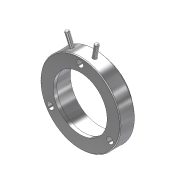
# Autodesk Inventor part: Part38
Saved by Autodesk Inventor 2011 (Build 150239000, 239)
## iProperties
Created: 2012-04-09
Part Number: Part38
Material: Steel
Document SubType Name: Modeling
Designer: jhanson2
Density: 7.85 g/cm^3
Author: jhanson2
Autodesk Inventor part; units mm, degrees
ref_plane "YZ Plane" through (0, 0, 0) normal (1, 0, 0) x (0, 1, 0)
sketch "Sketch1" plane through (0, 0, 0) normal (0, 0, 1) x (1, 0, 0)
  circle A0 centre (0, 0) radius 26.1938
  circle A1 centre (0, 0) radius 38.8938
  dimension "d0" = 77.7875
  dimension "d1" = 12.7
  constraints: 2 centre point, 2 coincident
  measures "d0" diameter of A1
  measures "d1" radial gap between concentric circles of A1 A0
extrude "Extrusion1" add sketch "Sketch1" along normal blind 14.5288
sketch "Sketch2" plane through (0, 0, 0) normal (0, 0, -1) x (-1, 0, 0)
  circle A0 centre (0, 0) radius 38.8938 projected
  circle A1 centre (0, 0) radius 28.575
  circle A2 centre (0, 0) radius 33.3375
  dimension "d5" = 4.7625
  dimension "d41" = 5.5563
  constraints: 2 centre point, 2 coincident
  measures "d5" radial gap between concentric circles of A1 A2
  measures "d41" radial gap between concentric circles of A2 A0
extrude "Extrusion2" add sketch "Sketch2" along normal blind 4.5212 contours A2
chamfer "Chamfer1" distance 0.7874 angle 45 1 edges at (33.3375, 0, -4.5212)
extrude "Extrusion3" cut sketch "Sketch2" against normal blind 11.1125 contours A1
sketch "Sketch3" plane through (0, 0, 14.5288) normal (0, 0, 1) x (1, 0, 0)
  circle A0 centre (0, 0) radius 38.8938 projected
  circle A1 centre (0, 33.3375) radius 3.175
  line L0 (0, 33.3375) -> (0, 0) construction
  dimension "d14" = 33.3375
  dimension "d15" = 6.35
  constraints: 2 end point, 1 centre point, 1 vertical
  measures "d14" distance of L0.start L0.end
  measures "d15" diameter of A1
extrude "Extrusion4" cut sketch "Sketch3" against normal blind 10.414 contours A1
pattern_circular "Circular Pattern1" count 3 over 360 about axis through (0, 0, 0) along (0, 0, 1) of "Extrusion4"
fillet "Fillet2" radius 0.7874 2 edges at (-38.8938, 0, 14.5288) (-38.8938, 0, 0)
sketch "Sketch4" plane through (0, 0, 14.5288) normal (0, 0, 1) x (1, 0, 0)
  circle A0 centre (0, 0) radius 26.1938 projected
  circle A1 centre (0, 33.3375) radius 3.175 projected
  circle A2 centre (-28.8711, -16.6687) radius 3.175 projected
  circle A3 centre (28.8711, -16.6688) radius 3.175 projected
  circle A4 centre (0, 0) radius 38.1064 projected
  line L0 (0, 0) -> (0, 33.3375) construction
  line L1 (8.1747, 37.2192) -> (10.5126, 50.4781) construction
  line L2 (0, 0) -> (8.9493, 50.7538) construction
  line L3 (5.048, 37.7705) -> (7.3859, 51.0295) construction
  line L4 (7.3859, 51.0295) -> (10.5126, 50.4781) construction
  line L5 (-13.4151, 35.6669) -> (-18.4691, 47.5734) construction
  line L6 (-16.3125, 34.3669) -> (-21.3917, 46.3328) construction
  line L7 (-21.3917, 46.3328) -> (-18.4691, 47.5734) construction
  line L8 (-19.9304, 46.9531) -> (0, 0) construction
  circle A5 centre (0, 46.0375) radius 6.35 projected
  dimension "d29" = 3.175
  dimension "d31" = 3.175
  dimension "d33" = 10
  dimension "d34" = 23
  constraints: 18 end point, 4 perpendicular, 3 point on circle, 2 midpoint, 2 parallel, 1 coincident
  measures "d29" distance between parallel lines of L1 L3
  measures "d31" distance between parallel lines of L5 L6
  measures "d33" angle of L2 L0
  measures "d34" angle of L0 L8
sketch "Sketch5" plane through (0, 0, 0) normal (0, 0, -1) x (-1, 0, 0)
  circle A0 centre (0, 0) radius 33.3375 projected
  circle A1 centre (0, 0) radius 38.1064 projected
  line L0 (19.9304, 46.9531) -> (0, 0) construction
  line L1 (0, 0) -> (-8.9493, 50.7538) construction
ref_plane "Work Plane1" through (0, 0, 14.5288) normal (-0.9848078, 0.1736482, 0) x (0.1736482, 0.9848078, 0)
ref_plane "Work Plane2" through (-19.9304, 46.9531, 0) normal (-0.9205049, -0.3907311, 0) x (0.3907311, -0.9205049, 0)
sketch "Sketch6" plane through (0, 0, 14.5288) normal (-0.9848078, 0.1736482, 0) x (0.1736482, 0.9848078, 0)
  line L0 (26.1938, 3.4163) -> (28.575, 3.4163) projected
  line L1 (26.1938, 0) -> (26.1938, 3.4163) projected
  line L2 (38.1064, 0) -> (26.1938, 0) projected
  arc A0 (38.1064, 0) -> (38.8938, 0.7874) centre (38.1064, 0.7874) ccw projected
  line L3 (38.8938, 13.7414) -> (38.8938, 0.7874) projected
  arc A1 (38.8938, 13.7414) -> (38.1064, 14.5288) centre (38.1064, 13.7414) ccw projected
  line L4 (33.3375, 14.5288) -> (38.1064, 14.5288) projected
  line L5 (33.3375, 18.2626) -> (33.3375, 14.5288) projected
  line L6 (32.5501, 19.05) -> (33.3375, 18.2626) projected
  line L7 (-33.3375, 18.2626) -> (-32.5501, 19.05) projected
  line L8 (-33.3375, 14.5288) -> (-33.3375, 18.2626) projected
  line L9 (-38.1064, 14.5288) -> (-33.3375, 14.5288) projected
  arc A2 (-38.1064, 14.5288) -> (-38.8938, 13.7414) centre (-38.1064, 13.7414) ccw projected
  line L10 (-38.8938, 0.7874) -> (-38.8938, 13.7414) projected
  arc A3 (-38.8938, 0.7874) -> (-38.1064, 0) centre (-38.1064, 0.7874) ccw projected
  line L11 (-26.1938, 0) -> (-38.1064, 0) projected
  line L12 (-26.1938, 3.4163) -> (-26.1938, 0) projected
  line L13 (-28.575, 3.4163) -> (-26.1938, 3.4163) projected
  line L14 (-38.8938, 5.28) -> (50.8, 5.28)
  line L15 (50.8, 5.28) -> (50.8, 7.2644)
  line L16 (-38.8938, 7.2644) -> (-38.8938, 5.28)
  arc A4 (50.8, 5.28) -> (52.7844, 7.2644) centre (50.8, 7.2644) ccw
  line L17 (50.8, 7.2644) -> (52.7844, 7.2644)
  line L18 (50.8, 7.2644) -> (-38.8938, 7.2644)
  line L19 (-38.8938, 7.2644) -> (35.5918, 7.2644)
  line L20 (35.5918, 7.2644) -> (35.5918, 5.28)
  line L21 (35.5918, 5.28) -> (-38.8938, 5.28)
  line L22 (-38.8938, 5.28) -> (-38.8938, 7.2644)
  line L23 (-26.1938, 1.7081) -> (26.1938, 1.7082) construction
  line L24 (0, 1.7081) -> (0, 14.5288) construction
  line L25 (28.575, 3.4163) -> (28.575, 19.05) projected
  line L26 (28.575, 19.05) -> (32.5501, 19.05) projected
  line L27 (-32.5501, 19.05) -> (-28.575, 19.05) projected
  line L28 (-28.575, 19.05) -> (-28.575, 3.4163) projected
  dimension "d35" = 3.9688
  dimension "d42" = 50.8
  constraints: 22 end point, 4 midpoint, 3 horizontal, 3 parallel, 3 perpendicular, 2 point on circle, 1 centre point, 1 collinear, 1 point on line, 1 tangent
  measures "d35" diameter of L14 L18
  measures "d42" distance from line of L24 L15.end
revolve "Revolution1" add sketch "Sketch6" angle 360 about axis through (8.8213, 50.0282, 7.2644) along (-0.1736482, -0.9848078, 0) contours L20 L18 L3 L14 | L3 L18 L15 L14 | L15 L17 A4
sketch "Sketch7" plane through (-19.9304, 46.9531, 0) normal (-0.9205049, -0.3907311, 0) x (0.3907311, -0.9205049, 0)
  line L0 (24.8142, 11.1125) -> (22.4329, 11.1125) projected
  line L1 (24.8142, 14.5288) -> (24.8142, 11.1125) projected
  line L2 (12.9016, 14.5288) -> (24.8142, 14.5288) projected
  arc A0 (12.9016, 14.5288) -> (12.1142, 13.7414) centre (12.9016, 13.7414) ccw projected
  line L3 (12.1142, 0.7874) -> (12.1142, 13.7414) projected
  arc A1 (12.1142, 0.7874) -> (12.9016, 0) centre (12.9016, 0.7874) ccw projected
  line L4 (17.6704, 0) -> (12.9016, 0) projected
  line L5 (17.6704, -3.7338) -> (17.6704, 0) projected
  line L6 (18.4578, -4.5212) -> (17.6704, -3.7338) projected
  line L7 (84.3454, -3.7338) -> (83.558, -4.5212) projected
  line L8 (84.3454, 0) -> (84.3454, -3.7338) projected
  line L9 (89.1143, 0) -> (84.3454, 0) projected
  arc A2 (89.1143, 0) -> (89.9017, 0.7874) centre (89.1143, 0.7874) ccw projected
  line L10 (89.9017, 13.7414) -> (89.9017, 0.7874) projected
  arc A3 (89.9017, 13.7414) -> (89.1143, 14.5288) centre (89.1143, 13.7414) ccw projected
  line L11 (77.2017, 14.5288) -> (89.1143, 14.5288) projected
  line L12 (77.2017, 11.1125) -> (77.2017, 14.5288) projected
  line L13 (79.5829, 11.1125) -> (77.2017, 11.1125) projected
  line L14 (89.9017, 7.2644) -> (0.2079, 7.2644)
  line L15 (0.2079, 7.2644) -> (0.2079, 9.2488)
  line L16 (0.2079, 9.2488) -> (89.9017, 9.2488)
  line L17 (89.9017, 9.2488) -> (89.9017, 7.2644)
  line L18 (89.9017, 7.2644) -> (14.9633, 7.2644)
  line L19 (14.9633, 7.2644) -> (14.9633, 9.2488)
  line L20 (14.9633, 9.2488) -> (89.9017, 9.2488)
  line L21 (89.9017, 9.2488) -> (89.9017, 7.2644)
  line L22 (0.2079, 7.2644) -> (-1.7764, 7.2644)
  arc A4 (0.2079, 9.2488) -> (-1.7764, 7.2644) centre (0.2079, 7.2644) ccw
  line L23 (51.0079, 0) -> (51.0079, 17.9555) construction
  line L24 (22.4329, 11.1125) -> (22.4329, -4.5212) projected
  line L25 (22.4329, -4.5212) -> (18.4578, -4.5212) projected
  line L26 (83.558, -4.5212) -> (79.5829, -4.5212) projected
  line L27 (79.5829, -4.5212) -> (79.5829, 11.1125) projected
  dimension "d39" = 3.9688
  dimension "d43" = 50.8
  constraints: 20 end point, 4 parallel, 4 perpendicular, 2 horizontal, 2 point on circle, 1 centre point, 1 collinear, 1 midpoint, 1 point on line, 1 tangent
  measures "d39" diameter of L16 L14
  measures "d43" distance from line of L23 L14.end
revolve "Revolution2" add sketch "Sketch7" angle 360 about axis through (15.197, -35.8019, 7.2644) along (-0.3907311, 0.9205049, 0) contours L19 L14 L3 L16 | L3 L14 L15 L16 | L15 L22 A4
equation "\"d31\" = d29"
body "Solid1"
